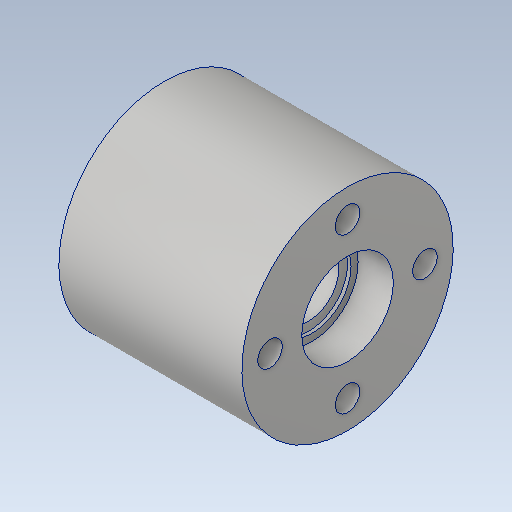
# Autodesk Inventor part: piasta_kola_przedniego_fi8
Saved by Autodesk Inventor 2020 (Build 240168000, 168)
## iProperties
Created: 2019-05-26
Part Number: piasta_kola_przedniego_fi8
Material: Aluminum 6061
Document SubType Name: Modeling
Designer: Besiu
Density: 2.7 g/cm^3
Appearance: Aluminum - Flat
Mass: 40.7813 g
Surface Area: 56.6076 cm^2
Volume: 15.1042 cm^3
Author: Besiu
Autodesk Inventor part; units mm, degrees
ref_plane "YZ Plane" through (0, 0, 0) normal (1, 0, 0) x (0, 1, 0)
sketch "Szkic1" plane through (0, 0, 0) normal (1, 0, 0) x (0, 1, 0)
  circle A0 centre (0, 0) radius 15
  dimension "d0" = 30
  constraints: 1 centre point, 1 coincident
  measures "d0" diameter of A0
extrude "Wyciągnięcie proste1" add sketch "Szkic1" along normal blind 26
sketch "Szkic2" plane through (26, 0, 0) normal (1, 0, 0) x (0, 0, -1)
  point P0 (0, 0)
  point P1 (0, 0)
  constraints: 1 coincident
hole "Otwór1" at (26, 0, 0) direction (-1, 0, 0) diameter 8.5 end through all
sketch "Szkic3" plane through (26, 0, 0) normal (1, 0, 0) x (0, 0, -1)
  point P0 (0, 0)
  point P1 (11, 0)
  point P2 (0, 11)
  point P3 (-11, 0)
  point P4 (0, -11)
  dimension "d10" = 11
  dimension "d13" = 360
  constraints: 1 horizontal alignment, 5 other
  measures "d10" distance of point (11, 0) point (0, 0)
hole "Otwór2" at (26, 0, -11) at (26, 11, 0) at (26, 0, 11) at (26, -11, 0) direction (-1, 0, 0) diameter 3.5 depth 26 tip angle 118
sketch "Szkic4" plane through (26, 0, 0) normal (1, 0, 0) x (0, 0, -1)
  line L0 (0, 0) -> (-10.6066, 10.6066)
  line L1 (0, 0) -> (15, 0) construction
  line L2 (0, 0) -> (10.6066, 10.6066)
  line L3 (0, 0) -> (15, 0) construction
  dimension "d22" = 15
  dimension "d23" = 135
  dimension "d24" = 15
  dimension "d25" = 45
  constraints: 8 end point, 2 equal length, 2 horizontal
  measures "d22" distance of L0.start L0.end
  measures "d23" angle of L1 L0
  measures "d24" distance of L0.start L2.end
  measures "d25" angle of L3 L2
ref_plane "Płaszczyzna konstrukcyjna1" through (26, 10.6066, 10.6066) normal (0, 0.7071, 0.7071) x (-1, 0, 0)
ref_plane "Płaszczyzna konstrukcyjna2" through (26, 10.6066, -10.6066) normal (0, 0.7071, -0.7071) x (-1, 0, 0)
sketch "Szkic7" plane through (0, 0, 0) normal (-1, 0, 0) x (0, 0, 1)
  circle A0 centre (0, 0) radius 6.5
  dimension "d42" = 13
  constraints: 1 centre point, 1 coincident
  measures "d42" diameter of A0
extrude "Wyciągnięcie proste2" cut sketch "Szkic7" against normal blind 5
sketch "Szkic13" plane through (5, 0, 0) normal (-1, 0, 0) x (0, 0, 1)
  circle A0 centre (0, 0) radius 5.5
  dimension "d80" = 11
  constraints: 1 centre point, 1 coincident
  measures "d80" diameter of A0
extrude "Wyciągnięcie proste5" cut sketch "Szkic13" against normal blind 0.5
sketch "Szkic14" plane through (26, 0, 0) normal (1, 0, 0) x (0, 0, -1)
  circle A0 centre (0, 0) radius 6.5
  dimension "d83" = 13
  constraints: 1 centre point, 1 coincident
  measures "d83" diameter of A0
extrude "Wyciągnięcie proste6" cut sketch "Szkic14" against normal blind 5
sketch "Szkic15" plane through (21, 0, 0) normal (1, 0, 0) x (0, 0, -1)
  circle A0 centre (0, 0) radius 5.5
  dimension "d86" = 11
  constraints: 1 centre point, 1 coincident
  measures "d86" diameter of A0
extrude "Wyciągnięcie proste7" cut sketch "Szkic15" against normal blind 0.5
equation "\"d0\" = radius"
equation "\"d16\" = d1"
equation "\"d20\" = d1"
equation "\"d22\" = 0.5 * radius"
equation "\"d24\" = d22"
equation "\"radius\" = 30"
equation "\"d1\" = 26"
